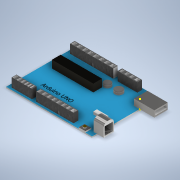
# Autodesk Inventor part: Arduino uno
Saved by Autodesk Inventor 2021 (Build 250183000, 183)
## iProperties
Created: 2021-07-03
Part Number: Arduino uno
Material: Generic
Document SubType Name: Modeling
Designer: ShivAni
Density: 1 g/cm^3
Appearance: Default
Author: ShivAni
Autodesk Inventor part; units mm, degrees
ref_plane "YZ Plane" through (0, 0, 0) normal (1, 0, 0) x (0, 1, 0)
ref_plane "XZ Plane" through (0, 0, 0) normal (0, 1, 0) x (-1, 0, 0)
ref_plane "XY Plane" through (0, 0, 0) normal (0, 0, 1) x (1, 0, 0)
sketch "Sketch1" plane through (0, 0, 0) normal (0, 1, 0) x (-1, 0, 0)
  line L0 (0.326, 37.5314) -> (68.326, 37.5314)
  line L1 (68.326, 37.5314) -> (68.326, -15.4686)
  line L2 (68.326, -15.4686) -> (0.326, -15.4686)
  line L3 (0.326, -15.4686) -> (0.326, 37.5314)
  point P0 (0, 0)
  dimension "d0" = 68
  dimension "d1" = 53
  constraints: 8 end point, 2 parallel, 1 horizontal, 1 perpendicular
  measures "d0" distance of L1.end L2.end
  measures "d1" distance of L0.end L1.end
extrude "Extrusion1" add sketch "Sketch1" along normal blind 1
sketch "Sketch2" plane through (0, 1, 0) normal (0, 1, 0) x (1, 0, 0)
  line L0 (-4.7532, 10.6227) -> (11.3789, 10.6227)
  line L1 (11.3789, 10.6227) -> (11.3789, 0)
  line L2 (11.3789, 0) -> (-4.7532, 0)
  line L3 (-4.7532, 0) -> (-4.7532, 10.6227)
  point P0 (0, 0)
  constraints: 8 end point, 2 parallel, 1 horizontal, 1 perpendicular
extrude "Extrusion2" add sketch "Sketch2" along normal blind 5
chamfer "Chamfer1" distance 0.5 angle 45 1 edges at (-4.7532, 1, -5.3113)
sketch "Sketch3" plane through (11.3789, 1, 0) normal (1, 0, 0) x (0, 0, -1)
  line L0 (0.7202, 1.1245) -> (9.7945, 1.1245)
  line L1 (9.7945, 1.1245) -> (9.7945, 3.9332)
  line L2 (9.7945, 3.9332) -> (0.7202, 3.9332)
  line L3 (0.7202, 3.9332) -> (0.7202, 1.1245)
  point P0 (0, -1)
  constraints: 8 end point, 2 parallel, 1 horizontal, 1 perpendicular
extrude "Extrusion3" cut sketch "Sketch3" against normal blind 15
sketch "Sketch4" plane through (0, 1, 0) normal (0, 1, 0) x (1, 0, 0)
  line L0 (-2.7772, -25.7946) -> (5.2178, -25.7946)
  line L1 (5.2178, -25.7946) -> (5.2178, -33.8739)
  line L2 (5.2178, -33.8739) -> (-2.7772, -33.8739)
  line L3 (-2.7772, -33.8739) -> (-2.7772, -25.7946)
  point P0 (0, 0)
  constraints: 8 end point, 2 parallel, 1 horizontal, 1 perpendicular
extrude "Extrusion4" add sketch "Sketch4" along normal blind 10
fillet "Fillet1" radius 3.175 2 edges at (1.2203, 11, 33.8739) (1.2203, 11, 25.7946)
sketch "Sketch5" plane through (5.2178, 1, 33.8739) normal (1, 0, 0) x (0, 0, -1)
  line L0 (0.8258, 1.006) -> (7.2858, 1.006)
  line L1 (7.2858, 1.006) -> (7.2858, 7.466)
  line L2 (7.2858, 7.466) -> (0.8258, 7.466)
  line L3 (0.8258, 7.466) -> (0.8258, 1.006)
  point P0 (33.8739, -1)
  constraints: 8 end point, 2 parallel, 1 horizontal, 1 perpendicular
extrude "Extrusion5" cut sketch "Sketch5" against normal blind 6.5
sketch "Sketch6" plane through (0, 1, 0) normal (0, 1, 0) x (1, 0, 0)
  point P0 (0, 0)
sketch "Sketch7" plane through (0, 1, 0) normal (0, 1, 0) x (1, 0, 0)
  point P0 (0, 0)
sketch "Sketch8" plane through (0, 1, 0) normal (0, 1, 0) x (1, 0, 0)
  line L0 (-68.326, -37.5314) -> (-0.326, -37.5314) projected
  line L1 (-10.8994, -32.9215) -> (-5.6284, -32.9215)
  line L2 (-5.6284, -32.9215) -> (-5.6284, -37.5314)
  line L3 (-5.6284, -37.5314) -> (-10.8994, -37.5314)
  line L4 (-10.8994, -37.5314) -> (-10.8994, -32.9215)
  point P0 (0, 0)
  constraints: 8 end point, 2 parallel, 1 horizontal, 1 perpendicular, 1 point on line
extrude "Extrusion6" add sketch "Sketch8" along normal blind 1
sketch "Sketch9" plane through (0, 2, 0) normal (0, 1, 0) x (1, 0, 0)
  circle A0 centre (-8.2639, -35.3337) radius 1.1219
  point P0 (0, 0)
  constraints: 1 centre point
extrude "Extrusion7" add sketch "Sketch9" along normal blind 1
sketch "Sketch10" plane through (0, 1, 0) normal (0, 1, 0) x (1, 0, 0)
  line L0 (-65.5808, -32.0709) -> (-49.5737, -32.0709)
  line L1 (-49.5737, -32.0709) -> (-49.5737, -35.8302)
  line L2 (-49.5737, -35.8302) -> (-65.5808, -35.8302)
  line L3 (-65.5808, -35.8302) -> (-65.5808, -32.0709)
  line L4 (-46.2996, -32.0709) -> (-16.7108, -32.0709)
  line L5 (-16.7108, -32.0709) -> (-16.7108, -35.8302)
  line L6 (-16.7108, -35.8302) -> (-46.2996, -35.8302)
  line L7 (-46.2996, -35.8302) -> (-46.2996, -32.0709)
  line L8 (-65.5808, 14.0099) -> (-31.5052, 14.0099)
  line L9 (-31.5052, 14.0099) -> (-31.5052, 10.3719)
  line L10 (-31.5052, 10.3719) -> (-65.5808, 10.3719)
  line L11 (-65.5808, 10.3719) -> (-65.5808, 14.0099)
  line L12 (-28.1098, 14.0099) -> (-12.4665, 14.0099)
  line L13 (-12.4665, 14.0099) -> (-12.4665, 10.3719)
  line L14 (-12.4665, 10.3719) -> (-28.1098, 10.3719)
  line L15 (-28.1098, 10.3719) -> (-28.1098, 14.0099)
  point P0 (0, 0)
  constraints: 32 end point, 8 parallel, 5 point on line, 4 horizontal, 4 perpendicular
extrude "Extrusion8" add sketch "Sketch10" along normal blind 7
sketch "Sketch11" plane through (0, 8, 0) normal (0, 1, 0) x (1, 0, 0)
  point P0 (0, 0)
sketch "Sketch12" plane through (0, 1, 0) normal (0, 1, 0) x (1, 0, 0)
  line L0 (-62.7472, 0) -> (-30.0328, 0)
  line L1 (-30.0328, 0) -> (-30.0328, -6.8378)
  line L2 (-30.0328, -6.8378) -> (-62.7472, -6.8378)
  line L3 (-62.7472, -6.8378) -> (-62.7472, 0)
  point P0 (0, 0)
  constraints: 8 end point, 2 parallel, 1 horizontal, 1 perpendicular
extrude "Extrusion9" add sketch "Sketch12" along normal blind 6
sketch "Sketch13" plane through (0, 1, 0) normal (0, 1, 0) x (1, 0, 0)
  circle A0 centre (-29.139, 3.4413) radius 2.7996
  circle A1 centre (-20.2007, 3.4413) radius 3.1284
  point P0 (0, 0)
  constraints: 2 centre point
extrude "Extrusion10" add sketch "Sketch13" along normal blind 2
sketch "Sketch14" plane through (0, 1, 0) normal (0, 1, 0) x (1, 0, 0)
  point P0 (0, 0)
sketch "Sketch15" plane through (0, 1, 0) normal (0, 1, 0) x (1, 0, 0)
  line L0 (-15.0164, -18.994) -> (-5.9887, -18.994)
  line L1 (-5.9887, -18.994) -> (-5.9887, -21.9436)
  line L2 (-5.9887, -21.9436) -> (-15.0164, -21.9436)
  line L3 (-15.0164, -21.9436) -> (-15.0164, -18.994)
  point P0 (0, 0)
  constraints: 8 end point, 2 parallel, 1 horizontal, 1 perpendicular
extrude "Extrusion11" add sketch "Sketch15" along normal blind 2
sketch "Sketch16" plane through (0, 8, 0) normal (0, 1, 0) x (1, 0, 0)
  point P0 (0, 0)
sketch "Sketch17" plane through (0, 8, 0) normal (0, 1, 0) x (1, 0, 0)
  point P0 (0, 0)
sketch "Sketch18" plane through (0, 8, 0) normal (0, 1, 0) x (1, 0, 0)
  line L0 (-45.9461, -32.5091) -> (-17.2073, -32.5091)
  line L1 (-17.2073, -32.5091) -> (-17.2073, -35.4675)
  line L2 (-17.2073, -35.4675) -> (-45.9461, -35.4675)
  line L3 (-45.9461, -35.4675) -> (-45.9461, -32.5091)
  line L4 (-44.355, -32.5091) -> (-44.355, -35.4675)
  line L5 (-42.3165, -32.5091) -> (-42.3165, -35.4675)
  line L6 (-40.2779, -32.5091) -> (-40.2779, -35.4675)
  line L7 (-38.3885, -32.5091) -> (-38.3885, -35.4675)
  line L8 (-36.6731, -32.5091) -> (-36.6731, -35.4675)
  line L9 (-34.6594, -32.5091) -> (-34.6594, -35.4675)
  line L10 (-32.7452, -32.5091) -> (-32.7452, -35.4675)
  line L11 (-30.9055, -32.5091) -> (-30.9055, -35.4675)
  line L12 (-28.842, -32.5091) -> (-28.842, -35.4675)
  line L13 (-26.9775, -32.5091) -> (-26.9775, -35.4675)
  line L14 (-25.0881, -32.5091) -> (-25.0881, -35.4675)
  line L15 (-23.1987, -32.5091) -> (-23.1987, -35.4675)
  line L16 (-21.4087, -32.5091) -> (-21.4087, -35.4675)
  line L17 (-19.6934, -32.5091) -> (-19.6934, -35.4675)
  point P0 (0, 0)
  constraints: 32 end point, 15 vertical, 1 parallel, 34 other
extrude "Extrusion12" cut sketch "Sketch18" against normal blind 7 contours L0 L4 L2 L3 | L0 L6 L2 L5 | L0 L8 L2 L7 | L0 L10 L2 L9 | L0 L12 L2 L11 | L0 L14 L2 L13 | L0 L16 L2 L15 | L0 L1 L2 L17
sketch "Sketch19" plane through (0, 8, 0) normal (0, 1, 0) x (1, 0, 0)
  line L0 (-65.3042, -32.3887) -> (-49.8579, -32.3887)
  line L1 (-49.8579, -32.3887) -> (-49.8579, -35.5948)
  line L2 (-49.8579, -35.5948) -> (-65.3042, -35.5948)
  line L3 (-65.3042, -35.5948) -> (-65.3042, -32.3887)
  line L4 (-63.6789, -32.3887) -> (-63.6789, -35.5948)
  line L5 (-61.99, -32.3887) -> (-61.99, -35.5948)
  line L6 (-60.4031, -32.3887) -> (-60.4031, -35.5948)
  line L7 (-58.9635, -32.3887) -> (-58.9635, -35.5948)
  line L8 (-57.4559, -32.3887) -> (-57.4559, -35.5948)
  line L9 (-56.1184, -32.3887) -> (-56.1184, -35.5948)
  line L10 (-54.7808, -32.3887) -> (-54.7808, -35.5948)
  line L11 (-53.6473, -32.3887) -> (-53.6473, -35.5948)
  line L12 (-52.5591, -32.3887) -> (-52.5591, -35.5948)
  line L13 (-51.5503, -32.3887) -> (-51.5503, -35.5948)
  line L14 (-50.6322, -32.3887) -> (-50.6322, -35.5948)
  point P0 (0, 0)
  constraints: 26 end point, 12 vertical, 1 parallel, 28 other
extrude "Extrusion13" cut sketch "Sketch19" against normal blind 7 contours L0 L4 L2 L3 | L0 L6 L2 L5 | L0 L8 L2 L7 | L0 L10 L2 L9 | L0 L12 L2 L11 | L0 L14 L2 L13
sketch "Sketch20" plane through (0, 1, 0) normal (0, 1, 0) x (1, 0, 0)
  line L0 (-55.91, -19.7296) -> (-31.8372, -19.7296) construction
  line L1 (-31.8372, -19.7296) -> (-31.8372, -22.9777) construction
  line L2 (-31.8372, -22.9777) -> (-55.91, -22.9777) construction
  line L3 (-55.91, -22.9777) -> (-55.91, -19.7296) construction
  point P0 (0, 0)
  constraints: 2 other
sketch "Sketch21" plane through (0, 8, 0) normal (0, 1, 0) x (1, 0, 0)
  line L0 (-65.1036, 13.5145) -> (-32.0202, 13.5145)
  line L1 (-32.0202, 13.5145) -> (-32.0202, 10.6777)
  line L2 (-32.0202, 10.6777) -> (-65.1036, 10.6777)
  line L3 (-65.1036, 10.6777) -> (-65.1036, 13.5145)
  line L4 (-62.9129, 13.5145) -> (-62.9129, 10.6777)
  line L5 (-60.9496, 13.5145) -> (-60.9496, 10.6777)
  line L6 (-58.797, 13.5145) -> (-58.797, 10.6777)
  line L7 (-56.4789, 13.5145) -> (-56.4789, 10.6777)
  line L8 (-54.4919, 13.5145) -> (-54.4919, 10.6777)
  line L9 (-52.3394, 13.5145) -> (-52.3394, 10.6777)
  line L10 (-50.2341, 13.5145) -> (-50.2341, 10.6777)
  line L11 (-48.0343, 13.5145) -> (-48.0343, 10.6777)
  line L12 (-45.6215, 13.5145) -> (-45.6215, 10.6777)
  line L13 (-43.4453, 13.5145) -> (-43.4453, 10.6777)
  line L14 (-41.2691, 13.5145) -> (-41.2691, 10.6777)
  line L15 (-39.2348, 13.5145) -> (-39.2348, 10.6777)
  line L16 (-37.1769, 13.5145) -> (-37.1769, 10.6777)
  line L17 (-34.9534, 13.5145) -> (-34.9534, 10.6777)
  point P0 (0, 0)
  constraints: 32 end point, 15 vertical, 1 parallel, 34 other
extrude "Extrusion14" cut sketch "Sketch21" against normal blind 7 contours L0 L4 L2 L3 | L0 L6 L2 L5 | L0 L8 L2 L7 | L0 L10 L2 L9 | L0 L12 L2 L11 | L0 L14 L2 L13 | L0 L16 L2 L15 | L0 L1 L2 L17
sketch "Sketch22" plane through (0, 8, 0) normal (0, 1, 0) x (1, 0, 0)
  line L0 (-27.265, 10.9849) -> (-13.4358, 10.9849)
  line L1 (-13.4358, 10.9849) -> (-13.4358, 13.5219)
  line L2 (-13.4358, 13.5219) -> (-27.265, 13.5219)
  line L3 (-27.265, 13.5219) -> (-27.265, 10.9849)
  line L4 (-25.5737, 10.9849) -> (-25.5737, 13.5219)
  line L5 (-23.4346, 10.9849) -> (-23.4346, 13.5219)
  line L6 (-21.5443, 10.9849) -> (-21.5443, 13.5219)
  line L7 (-19.5545, 10.9849) -> (-19.5545, 13.5219)
  line L8 (-17.5398, 10.9849) -> (-17.5398, 13.5219)
  line L9 (-15.6246, 10.9849) -> (-15.6246, 13.5219)
  point P0 (0, 0)
  constraints: 20 end point, 12 point on line, 7 perpendicular, 2 parallel, 1 horizontal
extrude "Extrusion15" cut sketch "Sketch22" against normal blind 7 contours L3 L2 L4 L0 | L5 L2 L6 L0 | L7 L2 L8 L0 | L9 L2 L1 L0
body "Solid1"
